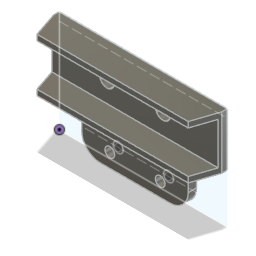
angel v1 (Autodesk Fusion 360 design; units mm, degrees)
Autodesk Fusion 360 part; units mm, degrees
sketch "Esquisse1" plane through (0, 0, 0) normal (0, 0, 1) x (1, 0, 0)
  line L0 (0, 0) -> (60, 0)
  line L1 (60, 0) -> (60, 36.5)
  line L2 (60, 36.5) -> (0, 36.5)
  line L3 (0, 36.5) -> (0, 0)
  line L4 (0, 5) -> (60, 5) construction
  line L5 (0, 33.5) -> (60, 33.5) construction
  circle A0 centre (21, 5) radius 1.75
  circle A1 centre (39, 5) radius 1.75
  dimension "d1" = 28.5
  dimension "d2" = 60
  dimension "d3" = 18
  dimension "d4" = 21
  dimension "d5" = 3.5
  dimension "d6" = 5
  dimension "d7" = 3
  constraint horizontal L0
  constraint vertical L1
  constraint horizontal L2
  constraint vertical L3
  constraint coincident L0.start L3.end
  constraint coincident L3 L4.start
  constraint coincident L1 L4.end
  constraint perpendicular L1 L4
  constraint coincident L3 L5.start
  constraint coincident L1 L5.end
  constraint perpendicular L1 L5
  constraint coincident L4 A0.centre
  constraint coincident L4 A1.centre
  constraint equal A0 A1
  measures "d1" distance of L4 L5
  measures "d2" distance of L1.end L2.end
  measures "d3" distance of A0.centre A1.centre
  measures "d4" distance of L1 A1.centre
  measures "d5" diameter of A0
  measures "d6" distance of L0 L4
  measures "d7" distance of L2 L5
extrude "Extrusion1" add sketch "Esquisse1" along normal blind 3
sketch "Esquisse2" plane through (0, 0, 3) normal (0, 0, 1) x (1, 0, 0)
  circle A0 centre (39, 5) radius 1.75
  circle A1 centre (21, 5) radius 1.75
  line L0 (0, 36.5) -> (0, 0)
  line L1 (0, 0) -> (60, 0)
  line L2 (60, 0) -> (60, 36.5)
  line L3 (60, 36.5) -> (0, 36.5)
  line L4 (0, 36.5) -> (60, 36.5)
  line L5 (60, 36.5) -> (60, 34.5)
  line L6 (60, 34.5) -> (0, 34.5)
  line L7 (0, 34.5) -> (0, 36.5)
  line L8 (0, 17.5) -> (60, 17.5)
  line L9 (60, 17.5) -> (60, 19.5)
  line L10 (60, 19.5) -> (0, 19.5)
  line L11 (0, 19.5) -> (0, 17.5)
  line L12 (60, 36.5) -> (0, 36.5)
  dimension "d10" = 15
  dimension "d11" = 2
  dimension "d12" = 2
  constraint horizontal L4
  constraint vertical L5
  constraint horizontal L6
  constraint vertical L7
  constraint coincident L2 L5.end
  constraint coincident L0 L3.end
  constraint horizontal L8
  constraint vertical L9
  constraint horizontal L10
  constraint vertical L11
  constraint coincident L2 L9.end
  constraint coincident L0 L8.start
  constraint collinear L4 L12
  measures "d10" distance of L6 L10
  measures "d11" distance of L8.end L9.end
  measures "d12" distance of L2.end L5.end
extrude "Extrusion2" add sketch "Esquisse2" along normal blind 8 contours L0 L2 L3 L4 L5 L6 L7 L12 | L0 L2 L8 L9 L10 L11
sketch "Esquisse3" plane through (0, 0, 3) normal (0, 0, 1) x (1, 0, 0)
  line L0 (0, 19.5) -> (60, 19.5)
  line L1 (60, 19.5) -> (60, 34.5)
  line L2 (60, 34.5) -> (0, 34.5)
  line L3 (0, 34.5) -> (0, 19.5)
  line L4 (0, 27) -> (60, 27) construction
  circle A0 centre (20, 27) radius 2.625
  circle A1 centre (40, 27) radius 2.625
  line L5 (0, 36.5) -> (0, 0)
  dimension "d17" = 15
  dimension "d18" = 60
  dimension "d19" = 20
  dimension "d20" = 20
  dimension "d21" = 5.25
  constraint midpoint L3 L4.start
  constraint midpoint L1 L4.end
  constraint coincident L4 A0.centre
  constraint coincident L4 A1.centre
  constraint equal A0 A1
  measures "d17" distance of L0 L2
  measures "d18" distance of L1.end L2.end
  measures "d19" distance of A0.centre L5
  measures "d20" distance of A0.centre A1.centre
  measures "d21" diameter of A0
chamfer "Chanfrein2" distance 3 distance2 9 4 edges at (0, 18.5, 11) (0, 35.5, 11) (60, 35.5, 11) (60, 18.5, 11) measured on face at (20, 18.8333, 11) measured on face at (20, 35.1667, 11) measured on face at (20, 35.1667, 11) measured on face at (20, 18.8333, 11)
extrude "Extrusion3" cut sketch "Esquisse3" against normal blind 8 contours A0 | A1
sketch "Esquisse5" plane through (0, 0, 3) normal (0, 0, 1) x (1, 0, 0)
  line L0 (59.6667, 0) -> (59.6667, 17.5)
  line L1 (59.6667, 17.5) -> (0.3333, 17.5)
  line L2 (0.3333, 17.5) -> (0.3333, 0)
  line L3 (0.3333, 0) -> (59.6667, 0)
  circle A0 centre (39, 5) radius 1.75
  circle A1 centre (21, 5) radius 1.75
  line L4 (11, 0) -> (-11.5098, 0)
  line L5 (-11.5098, 0) -> (-11.5098, 17.5)
  line L6 (-11.5098, 17.5) -> (11, 17.5)
  line L7 (11, 17.5) -> (11, 0)
  line L8 (49, 0) -> (81.8509, 0)
  line L9 (81.8509, 0) -> (81.8509, 17.5)
  line L10 (81.8509, 17.5) -> (49, 17.5)
  line L11 (49, 17.5) -> (49, 0)
  point P0 (21, 5)
  point P1 (39, 5)
  dimension "d31" = 10
  dimension "d32" = 10
  constraint horizontal L4
  constraint vertical L5
  constraint horizontal L6
  constraint vertical L7
  constraint coincident L3 L4.start
  constraint horizontal L8
  constraint vertical L9
  constraint horizontal L10
  constraint vertical L11
  constraint coincident L3 L8.start
  constraint collinear L1 L6
  constraint collinear L1 L10
  measures "d31" distance of L7 P0
  measures "d32" distance of L11 P1
extrude "Extrusion5" cut sketch "Esquisse5" against normal blind 20 contours L0 L1 L3 L8 L10 L11 | L0 L8 L9 L10 | L1 L2 L3 L4 L6 L7 | L2 L4 L5 L6
fillet "Congé2" radius 6.5 4 edges at (11, 17.5, 1.5) (11, 0, 1.5) (49, 17.5, 1.5) (49, 0, 1.5)
equation "d4 = ( d2 - d3 ) / 2"
equation "d19 = d18 / 3"
equation "d20 = d19"
